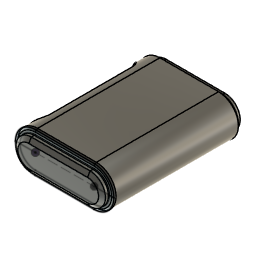
Router Case (Autodesk Fusion 360 archive; units mm, degrees)
design "Router"
Autodesk Fusion 360 part; units mm, degrees
note: some values were not read from the file. Chosen so that the rebuilt part matches the saved one: a side; which pieces of a blend or face edit are solid.
sketch "Sketch1" plane through (0, 0, 0) normal (0, 1, 0) x (1, 0, 0)
  line L0 (0, -18.1) -> (53.8, -18.1)
  arc A0 (53.8, -18.1) -> (53.8, 18.1) centre (53.8, 0) ccw
  line L1 (53.8, 18.1) -> (0, 18.1)
  arc A1 (0, 18.1) -> (0, -18.1) centre (0, 0) ccw
  line L2 (0, 0) -> (53.8, 0) construction
  line L3 (0, 0) -> (-18.1, 0)
  line L4 (53.8, 0) -> (71.9, 0)
  line L5 (53.8, 14.1) -> (0, 14.1)
  arc A2 (0, 14.1) -> (0, -14.1) centre (0, 0) ccw
  line L6 (0, -14.1) -> (53.8, -14.1)
  arc A3 (53.8, -14.1) -> (53.8, 14.1) centre (53.8, 0) ccw
  dimension "d1" = 36.2
  dimension "d2" = 90
  dimension "d6" = -4
  constraint tangent L0 A0
  constraint tangent A0 L1
  constraint parallel L0 L1
  constraint tangent L1 A1
  constraint tangent L0 A1
  constraint horizontal L2
  constraint coincident A1.centre L2.start
  constraint midpoint A1 L3.end
  constraint coincident A0.centre L2.end
  constraint midpoint A0 L4.end
  measures "d1" diameter of A0
  measures "d2" distance of L3.end L4.end
extrude "Extrude1" add sketch "Sketch1" along normal blind 116 makes body 1
ref_plane "WorkPlane1" through (0, 58, 0) normal (0, 1, 0) x (0, 0, 1)
extrude "Extrude2" add sketch "Sketch1" against normal blind 6 separate body contours L5 A2 L6 A3 makes body 2
sketch "Sketch2" plane through (0, 0, 18.1) normal (0, 0, 1) x (-1, 0, 0)
  line L0 (0, 0) -> (-53.8, 0)
  line L1 (-53.8, 0) -> (-53.8, -116)
  line L2 (-53.8, -116) -> (0, -116)
  line L3 (0, -116) -> (0, 0)
  line L4 (0, 0) -> (0, -116)
  line L5 (0, -58) -> (-47.3053, -58)
  line L6 (7, -58) -> (7, -105.5)
  line L7 (7, -105.5) -> (47, -105.5)
  line L8 (47, -105.5) -> (47, -10.5)
  line L9 (47, -10.5) -> (7, -10.5)
  line L10 (7, -10.5) -> (7, -58)
  dimension "d9" = 95
  dimension "d10" = 40
  dimension "d11" = 7
  constraint coincident L0.start L3.end
  constraint coincident L2.end L3.start
  constraint midpoint L3 L5.start
  constraint perpendicular L4 L5
  constraint coincident L5 L6.start
  constraint perpendicular L5 L6
  constraint perpendicular L3 L7
  constraint perpendicular L5 L8
  constraint perpendicular L3 L9
  constraint perpendicular L9 L10
  constraint equal L6 L10
  measures "d9" distance of L7 L9
  measures "d10" distance of L8 L10
  measures "d11" distance of L4 L6
extrude "Extrude3" cut sketch "Sketch2" against normal blind 50 contours L6 L7 L8 L9 L10 bodies 1
fillet "Fillet1" radius 11 2 edges at (-7, 105.5, 0) (-7, 10.5, 0) on bodies 1
chamfer "Chamfer1" distance 4 angle 30 4 edges at (26.9, -6, 14.1) (-14.1, -6, 0) (26.9, -6, -14.1) (67.9, -6, 0) measured on face at (17.9333, -4, 14.1) measured on face at (-8.716, -4, -11.0833) measured on face at (35.8667, -4, -14.1) measured on face at (55.1403, -4, -14.0362) on bodies 2
chamfer "Chamfer2" distance 1 angle 45 4 edges at (26.9, 0, 14.1) (67.9, 0, 0) (26.9, 0, -14.1) (-14.1, 0, 0) on bodies 2
chamfer "Chamfer3" distance 2 angle 45 8 edges at (26.9, 0, 18.1) (71.9, 0, 0) (26.9, 0, -18.1) (-18.1, 0, 0) (26.9, 116, 18.1) (71.9, 116, 0) (26.9, 116, -18.1) (-18.1, 116, 0) on bodies 1
fillet "Fillet2" radius 0.5 8 edges at (-12.6949, 11.8643, 12.9005) (-18.1, 10.5, 0) (-12.6949, 11.8643, -12.9005) (-7, 58, -16.6916) (-12.6949, 104.1357, -12.9005) (-18.1, 105.5, 0) (-12.6949, 104.1357, 12.9005) (-7, 58, 16.6916) on bodies 1
mirror "Mirror1" about plane through (0, 58, 0) normal (0, 1, 0) of bodies 2 makes body 3
equation "d5 = ( 116 / 2 ) * 1 mm"
equation "d7 = ( -( 128 - 116 ) / 2 ) * 1 mm"
